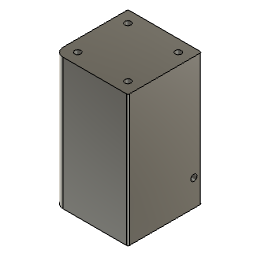
Leg_Extension_Front_Left (Autodesk Fusion 360 design; units mm, degrees)
Autodesk Fusion 360 part; units mm, degrees
sketch "Skizze1" plane through (0, 0, 0) normal (0, 0, 1) x (1, 0, 0)
  line L0 (0, 0) -> (50.5, 0)
  line L1 (50.5, 0) -> (50.5, 50.5)
  line L2 (50.5, 50.5) -> (0, 50.5)
  line L3 (0, 50.5) -> (0, 0)
  line L4 (0, 0) -> (0, -25)
  line L5 (0, 0) -> (5, 0)
  line L6 (5, 0) -> (5, -30)
  line L7 (5, 0) -> (8.5, 0)
  line L8 (8.5, 0) -> (8.5, -30)
  line L9 (8.5, 0) -> (13.5, 0)
  line L10 (13.5, 0) -> (13.5, -25)
  line L11 (0, -25) -> (5, -30)
  line L12 (8.5, -30) -> (13.5, -25)
  line L13 (25.25, 50.5) -> (25.25, 0)
  line L14 (42.5, 42.5) -> (8, 42.5)
  line L15 (8, 42.5) -> (8, 8)
  line L16 (8, 8) -> (42.5, 8)
  line L17 (42.5, 8) -> (42.5, 42.5)
  line L18 (42.5, 42.5) -> (8, 8) construction
  line L19 (8, 42.5) -> (42.5, 8) construction
  circle A0 centre (25.25, 25.25) radius 12.7
  point P0 (25.25, 25.25)
  dimension "d1" = 50.5
  dimension "d2" = 50.5
  dimension "d3" = 25
  dimension "d4" = 5
  dimension "d5" = 30
  dimension "d6" = 3.5
  dimension "d7" = 30
  dimension "d8" = 5
  dimension "d9" = 25
  dimension "d10" = 34.5
  dimension "d11" = 34.5
  dimension "d12" = 25.4
  constraint horizontal L0
  constraint vertical L1
  constraint horizontal L2
  constraint vertical L3
  constraint coincident L0.start L3.end
  constraint perpendicular L0 L4
  constraint perpendicular L4 L5
  constraint perpendicular L0 L6
  constraint perpendicular L6 L7
  constraint perpendicular L7 L8
  constraint perpendicular L8 L9
  constraint perpendicular L0 L10
  constraint midpoint L2 L13.start
  constraint midpoint L0 L13.end
  constraint perpendicular L14 L15
  constraint parallel L14 L16
  constraint parallel L15 L17
  constraint horizontal L14
  constraint coincident L18 P0
  constraint coincident L19 P0
  constraint midpoint L13 P0
  constraint coincident P0 A0.centre
  measures "d1" distance of L0.start L0.end
  measures "d2" distance of L0.start L2.end
  measures "d3" distance of L0.start L4.end
  measures "d4" distance of L0.start L5.end
  measures "d5" distance of L5.end L6.end
  measures "d6" distance of L5.end L7.end
  measures "d7" distance of L7.end L8.end
  measures "d8" distance of L7.end L9.end
  measures "d9" distance of L9.end L10.end
  measures "d10" distance of L15.end L16.end
  measures "d11" distance of L14.end L15.end
  measures "d12" diameter of A0
extrude "Extrusion1" add sketch "Skizze1" against normal blind 90 contours L0 L2 L3 L5 L7 L9 L13 L14 L15 L16 | L0 L1 L2 L13 L14 L16 L17 | L13 L14 L16 L17 A0 | L13 L14 L15 L16 A0 | L13 A0 | L13 A0
extrude "Extrusion2" cut sketch "Skizze1" against normal blind 15 contours L13 A0 | L13 A0
chamfer "Fase1" distance 2.5 distance2 15 1 edges at (13.4094, 29.8425, 0) measured on face at (25.5664, 4.1952, 0)
hole "Bohrung1" at (42.5, 42.5, 0) at (42.5, 8, 0) at (8, 8, 0) at (8, 42.5, 0) direction (0, 0, -1) diameter 8.8 depth 82 tip angle 180
hole "Bohrung2" at (8, 42.5, -82) direction (0, 0, -1) diameter 4.2 depth 82 tip angle 180 countersink diameter 8.6 countersink angle 90
hole "Bohrung3" at (42.5, 42.5, -82) direction (0, 0, -1) diameter 4.2 depth 82 tip angle 180 countersink diameter 8.6 countersink angle 90
hole "Bohrung4" at (42.5, 8, -82) direction (0, 0, -1) diameter 4.2 depth 82 tip angle 180 countersink diameter 8.6 countersink angle 90
hole "Bohrung5" at (8, 8, -82) direction (0, 0, -1) diameter 4.2 depth 82 tip angle 180 countersink diameter 8.6 countersink angle 90
ref_plane "Arbeitsebene1" through (8.5, -15, 0) normal (-1, 0, 0) x (0, -1, 0)
ref_plane "Arbeitsebene2" through (5, -15, 0) normal (-1, 0, 0) x (0, -1, 0)
sketch "Skizze2" plane through (5, -15, 0) normal (-1, 0, 0) x (0, 1, 0)
  line L0 (15, 0) -> (15, 30)
  line L1 (15, 0) -> (-15, 0)
  arc A0 (15, 30) -> (-15, 0) centre (15, 0) ccw
  dimension "d44" = 30
  dimension "d45" = 30
  constraint vertical L0
  constraint perpendicular L0 L1
  measures "d44" distance of L0.start L0.end
  measures "d45" distance of L0.start L1.end
sketch "Skizze3" plane through (8.5, -15, 0) normal (-1, 0, 0) x (0, 1, 0)
  line L0 (15, 0) -> (-15, 0)
  line L1 (15, 0) -> (15, 30)
  arc A0 (15, 30) -> (-15, 0) centre (15, 0) ccw
  dimension "d46" = 30
  dimension "d47" = 30
  constraint horizontal L0
  constraint perpendicular L0 L1
  measures "d46" distance of L0.start L0.end
  measures "d47" distance of L0.start L1.end
sketch "Skizze4" plane through (0, 0, 0) normal (-1, 0, 0) x (0, -1, 0)
  line L0 (0, 0) -> (-50.5, 0)
  line L1 (-50.5, 0) -> (-50.5, -90)
  line L2 (-50.5, -90) -> (0, -90)
  line L3 (0, -90) -> (0, 0)
  line L4 (0, 0) -> (10, 0)
  line L5 (10, 0) -> (10, -10)
  line L6 (10, -10) -> (0, -10)
  line L7 (0, -10) -> (0, 0)
  dimension "d54" = 10
  dimension "d55" = 10
  constraint horizontal L4
  constraint vertical L5
  constraint horizontal L6
  constraint vertical L7
  measures "d54" distance of L0.start L4.end
  measures "d55" distance of L0.start L6.end
sketch "Skizze6" plane through (0, 0, 0) normal (0, -1, 0) x (1, 0, 0)
  line L0 (0, 0) -> (0, -90)
  line L1 (0, -90) -> (50.5, -90)
  line L2 (50.5, -90) -> (50.5, 0)
  line L3 (50.5, 0) -> (0, 0)
  line L4 (50.5, 0) -> (42.1, 0)
  line L5 (42.1, 0) -> (42.1, -29.9)
  line L6 (42.1, -29.9) -> (50.5, -29.9)
  line L7 (50.5, -29.9) -> (50.5, 0)
  line L8 (50.5, 0) -> (42.1, 0)
  line L9 (42.1, 0) -> (42.1, -9.1)
  line L10 (42.1, -9.1) -> (50.5, -9.1)
  line L11 (50.5, -9.1) -> (50.5, 0)
  dimension "d64" = 8.4
  dimension "d65" = 29.9
  dimension "d66" = 9.1
  constraint horizontal L4
  constraint vertical L5
  constraint horizontal L6
  constraint vertical L7
  constraint coincident L2.end L3.start
  constraint horizontal L8
  constraint vertical L9
  constraint horizontal L10
  constraint vertical L11
  measures "d64" distance of L2.end L4.end
  measures "d65" distance of L2.end L6.end
  measures "d66" distance of L2.end L10.end
hole "Bohrung7" at (42.1, 0, -9.1) at (42.1, 0, -29.9) direction (0, 1, 0) diameter 4.2 depth 9 tip angle 180
sketch "Skizze7" plane through (50.5, 0, 0) normal (1, 0, 0) x (0, 1, 0)
  line L0 (50.5, 0) -> (0, 0)
  line L1 (0, 0) -> (0, -90)
  line L2 (0, -90) -> (50.5, -90)
  line L3 (50.5, -90) -> (50.5, 0)
  line L4 (0, 0) -> (5.3, 0)
  line L5 (5.3, 0) -> (5.3, -18.1)
  line L6 (5.3, -18.1) -> (0, -18.1)
  line L7 (0, -18.1) -> (0, 0)
  dimension "d72" = 18.1
  dimension "d73" = 5.3
  constraint horizontal L4
  constraint vertical L5
  constraint horizontal L6
  constraint vertical L7
  constraint coincident L0.end L1.start
  measures "d72" distance of L0.end L6.end
  measures "d73" distance of L0.end L4.end
hole "Bohrung8" at (50.5, 5.3, -18.1) direction (-1, 0, 0) diameter 4.2 depth 13 tip angle 180
move_body "Verschieben1" bodies 1 to x (-1, 0, 0) y (0, 1, 0) z (0, 0, -1) at (101, 0, 0)
move_body "Verschieben2" bodies 1 to x (1, 0, 0) y (0, 1, 0) z (0, 0, 1) at (-101, -50.5, 0)
move_body "Verschieben3" bodies 1 to x (-1, 0, 0) y (0, -1, 0) z (0, 0, 1) at (0, 0, 0)
fillet "Fillet4" radius 6 1 edges at (0, 0, 45)
fillet "Fillet5" radius 1 3 edges at (50.5, 0, 45) (50.5, 50.5, 45) (0, 50.5, 45)
